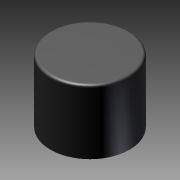
# Autodesk Inventor part: SB40-plunger
Saved by Autodesk Inventor 2014 (Build 180170000, 170)
## iProperties
Category: PARTsolutions
Company: NKKSWITCHES
Created: 2013-12-28
Part Number: SB40-plunger
Catalog Web Link: www.cadenas.de
Description: SB4011 Series - 3 Amp Momentary Pushbuttons -plunger-
Vendor: NKKSWITCHES
Document SubType Name: Modeling
Designer: PARTuser1
Manufacturer: NKKSWITCHES
Density: 1 g/cm^3
Material: Generic
Appearance: RGB(0.00000000000000,0.00000000000000,0.00000000000000)
PSOL_IDENT_0: {$CADENAS_DATA\23d-libs\nkkswitches\pushbuttons\sb4011\parts\sb4011_plunger.prj},220 {VTYP=3D},{NB=S
PSOL_IDENT_1: B40-plunger},{LINA=SB40-plunger},{NN=SB4011 Series - 3 Amp Momentary Pushbuttons -plunger},{DATE=17.
PSOL_IDENT_2: 02.2009 10:23:06},{GEOMDATE=16.02.2009 09:10:00},{VERSION=},{LINEID=10},{LINESUBID=-1},{WBVAR=PLNGRC
PSOL_IDENT_3: LR}  {NB=SB40-plunger},{LINA=SB40-plunger},{KT=DUMMY},{PN=SB40},{SRS=SB40},{PLNGRCLR=},{PLNGRCLRALG=
PSOL_IDENT_4: 0.00,0.00,0.00,0.00 }
CNS_NN: SB4011 Series - 3 Amp Momentary Pushbuttons -plunger
CNS_NB: SB40-plunger
CNS_NBSYN: $PN.-plunger
CNS_LINA: SB40-plunger
CNS_PN: SB40
CNS_SRS: SB40
CNS_PLNGRCLR: Black
CNS_PLNGRCLRALG: 0.00,0.00,0.00,0.00
SUPPLIER: NKKSWITCHES
ARTICLENO: SB40-plunger
BOMINFO: SB40-plunger
CREATOR: CADENAS GmbH
Title: SB40-plunger
Author: Cadenas PARTsolutions
Autodesk Inventor part; units mm, degrees
sketch "Sketch_2" plane through (0, 0, 0) normal (1, 0, 0) x (0, 1, 0)
  line L0 (-0.508, 0) -> (6.2992, 0)
  line L1 (6.2992, 0) -> (6.2992, -3.9497)
  arc A0 (6.0452, -4.2037) -> (6.2992, -3.9497) centre (6.0452, -3.9497) ccw
  line L2 (6.0452, -4.2037) -> (-0.508, -4.2037)
  line L3 (-0.508, -4.2037) -> (-0.508, 0)
  line L4 (-0.508, 0) -> (6.2992, 0)
  constraints: 10 end point, 2 point on circle, 1 centre point
revolve "Revolution1" add sketch "Sketch_2" angle 360 about axis through (0, -0.508, 0) along (0, -1, 0)
ref_plane "to_body_XY" through (0, 0, 0) normal (0, 1, 0) x (1, 0, 0)
ref_plane "to_body_YZ" through (0, 0, 0) normal (1, 0, 0) x (0, 0, -1)
ref_plane "to_body_ZX" through (0, 0, 0) normal (0, 0, -1) x (0, 1, 0)
ref_plane "to_cap_XY" through (0, 2.794, 0) normal (0, -1, 0) x (1, 0, 0)
ref_plane "to_cap_YZ" through (0, 2.794, 0) normal (1, 0, 0) x (0, 0, 1)
ref_plane "to_cap_ZX" through (0, 2.794, 0) normal (0, 0, 1) x (0, -1, 0)
body "Solid1"
